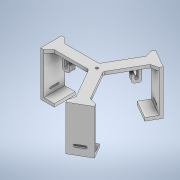
# Autodesk Inventor part: CalibrationRig_ver2
Saved by Autodesk Inventor 2022 (Build 260153000, 153)
## iProperties
Created: 2022-04-08
Part Number: CalibrationRig_ver2
Material: Generic
Document SubType Name: Modeling
Designer: victo
Density: 1 g/cm^3
Appearance: Default
Author: victo
Autodesk Inventor part; units mm, degrees
ref_plane "YZ Plane" through (0, 0, 0) normal (1, 0, 0) x (0, 1, 0)
ref_plane "XZ Plane" through (0, 0, 0) normal (0, 1, 0) x (-1, 0, 0)
ref_plane "XY Plane" through (0, 0, 0) normal (0, 0, 1) x (1, 0, 0)
sketch "Sketch1" plane through (0, 0, 0) normal (0, 1, 0) x (-1, 0, 0)
  line L0 (0, 0) -> (-20, 0)
  line L1 (0, 80) -> (-20, 80)
  line L2 (-20, 80) -> (-20, 120)
  line L3 (-20, 120) -> (0, 120)
  line L4 (0, 120) -> (6, 120)
  line L5 (6, 120) -> (6, 80)
  line L6 (6, 80) -> (0, 80)
  line L7 (-105.746, 18.9475) -> (-108.746, 13.7513)
  line L8 (-108.746, 13.7513) -> (-143.3871, 33.7513)
  line L9 (-143.3871, 33.7513) -> (-130.3871, 56.268)
  line L10 (-95.746, 36.268) -> (-108.746, 13.7513)
  line L11 (-95.746, 36.268) -> (-130.3871, 56.268)
  line L12 (-140.3871, 161.0525) -> (-143.3871, 166.2487)
  line L13 (-143.3871, 166.2487) -> (-108.746, 186.2487)
  line L14 (-108.746, 186.2487) -> (-95.746, 163.732)
  line L15 (-130.3871, 143.732) -> (-143.3871, 166.2487)
  line L16 (-130.3871, 143.732) -> (-95.746, 163.732)
  dimension "d12" = 40
  dimension "d13" = 6
  dimension "d15" = 6
  dimension "d16" = 40
  dimension "d18" = 6
  dimension "d19" = 40
  constraints: 34 end point, 2 horizontal, 2 perpendicular, 2 point on line, 1 collinear, 1 parallel, 1 vertical
  measures "d12" distance of L1.end L2.end
  measures "d13" distance of L3.end L4.end
  measures "d15" distance of L7.start L7.end
  measures "d16" distance of L7.end L8.end
  measures "d18" distance of L12.start L12.end
  measures "d19" distance of L12.end L13.end
extrude "Extrusion1" add sketch "Sketch1" along normal blind 6
sketch "Sketch2" plane through (0, 6, 0) normal (0, 1, 0) x (1, 0, 0)
  line L0 (-6, -80) -> (-6, -120) projected
  line L1 (20, -80) -> (-6, -80) projected
  line L2 (-6, -120) -> (0, -120)
  line L3 (0, -120) -> (0, -80)
  line L4 (0, -80) -> (-6, -80)
  line L5 (-6, -80) -> (-6, -120)
  line L6 (143.3871, -166.2487) -> (130.3871, -143.732) projected
  line L7 (95.746, -163.732) -> (108.746, -186.2487) projected
  line L8 (143.3871, -166.2487) -> (108.746, -186.2487)
  line L9 (108.746, -186.2487) -> (105.746, -181.0525)
  line L10 (105.746, -181.0525) -> (140.3871, -161.0525)
  line L11 (140.3871, -161.0525) -> (143.3871, -166.2487)
  line L12 (130.3871, -56.268) -> (143.3871, -33.7513) projected
  line L13 (143.3871, -33.7513) -> (108.746, -13.7513)
  line L14 (108.746, -13.7513) -> (105.746, -18.9475)
  line L15 (108.746, -13.7513) -> (95.746, -36.268) projected
  line L16 (143.3871, -33.7513) -> (108.746, -13.7513) projected
  line L17 (105.746, -18.9475) -> (140.3871, -38.9475)
  line L18 (143.3871, -33.7513) -> (140.3871, -38.9475)
  point P0 (0, 0)
  dimension "d22" = 6
  dimension "d23" = 6
  constraints: 24 end point, 8 perpendicular, 4 point on line, 2 parallel, 1 horizontal
  measures "d22" distance of L7.end L9.end
  measures "d23" distance of L13.end L14.end
extrude "Extrusion2" add sketch "Sketch2" along normal blind 80
sketch "Sketch3" plane through (0, 6, 120) normal (1, 0, 0) x (0, 0, -1)
  line L0 (0, 80) -> (40, 80) projected
  line L1 (40, -6) -> (40, 80) projected
  line L2 (0, 80) -> (40, 80)
  line L3 (40, 80) -> (40, 74)
  line L4 (40, 74) -> (0, 74)
  line L5 (0, 74) -> (0, 80)
  point P0 (120, -6)
  dimension "d26" = 6
  constraints: 8 end point, 2 parallel, 1 horizontal, 1 perpendicular, 1 point on line
  measures "d26" distance of L2.end L3.end
extrude "Extrusion3" add sketch "Sketch3" along normal blind 10
sketch "Sketch4" plane through (140.3871, 6, 38.9475) normal (-0.5, 0, 0.8660254) x (0.8660254, 0, 0.5)
  line L0 (0, 80) -> (-40, 80) projected
  line L1 (0, -6) -> (0, 80) projected
  line L2 (-40, 80) -> (0, 80)
  line L3 (0, 80) -> (0, 74)
  line L4 (0, 74) -> (-40, 74)
  line L5 (-40, 74) -> (-40, 80)
  point P0 (-141.0525, -6)
  dimension "d29" = 6
  constraints: 8 end point, 2 parallel, 1 horizontal, 1 perpendicular, 1 point on line
  measures "d29" distance of L2.end L3.end
extrude "Extrusion4" add sketch "Sketch4" along normal blind 10
sketch "Sketch5" plane through (105.746, 6, 181.0525) normal (-0.5, 0, -0.8660254) x (-0.8660254, 0, 0.5)
  line L0 (-40, 80) -> (0, 80) projected
  line L1 (0, 0) -> (0, 80) projected
  line L2 (-40, 80) -> (0, 80)
  line L3 (0, 80) -> (0, 74)
  line L4 (0, 74) -> (-40, 74)
  line L5 (-40, 74) -> (-40, 80)
  point P0 (1.0525, -6)
  dimension "d32" = 6
  constraints: 8 end point, 2 parallel, 1 horizontal, 1 perpendicular, 1 point on line
  measures "d32" distance of L2.end L3.end
extrude "Extrusion5" add sketch "Sketch5" along normal blind 10
chamfer "Chamfer1" distance 10 angle 45 6 edges at (100.746, 83, 27.6077) (135.3871, 83, 47.6077) (135.3871, 83, 152.3923) (100.746, 83, 172.3923) (10, 83, 120) (10, 83, 80)
sketch "Sketch6" plane through (135.3871, 6, 47.6077) normal (-0.5, 0, 0.8660254) x (0.8660254, 0, 0.5)
  line L0 (-30, 74) -> (-10, 74) projected
  line L1 (-10, 80) -> (-10, 74) projected
  line L2 (-30, 74) -> (-10, 74)
  line L3 (-10, 74) -> (-10, 80)
  line L4 (-10, 80) -> (-30, 80)
  line L5 (-30, 80) -> (-30, 74)
  point P0 (-141.0525, -6)
  constraints: 8 end point, 2 parallel, 1 horizontal, 1 perpendicular
extrude "Extrusion6" add sketch "Sketch6" along normal blind 90
sketch "Sketch7" plane through (10, 6, 120) normal (1, 0, 0) x (0, 0, -1)
  line L0 (10, 80) -> (0, 80) projected
  line L1 (30, 74) -> (40, 74) projected
  line L2 (10, 80) -> (30, 80)
  line L3 (30, 80) -> (30, 74)
  line L4 (30, 74) -> (10, 74)
  line L5 (10, 74) -> (10, 80)
  point P0 (120, -6)
  constraints: 8 end point, 2 parallel, 1 horizontal, 1 perpendicular
extrude "Extrusion7" add sketch "Sketch7" along normal through all
sketch "Sketch8" plane through (100.746, 6, 172.3923) normal (-0.5, 0, -0.8660254) x (-0.8660254, 0, 0.5)
  line L0 (-30, 80) -> (-40, 80) projected
  line L1 (-30, 74) -> (-10, 74) projected
  line L2 (-30, 80) -> (-10, 80)
  line L3 (-10, 80) -> (-10, 74)
  line L4 (-10, 74) -> (-30, 74)
  line L5 (-30, 74) -> (-30, 80)
  point P0 (1.0525, -6)
  constraints: 8 end point, 2 parallel, 1 horizontal, 1 perpendicular
extrude "Extrusion8" add sketch "Sketch8" along normal up to next
sketch "Sketch9" plane through (0, 86, 0) normal (0, 1, 0) x (1, 0, 0)
  line L0 (93.5914, -100) -> (113.5914, -100) construction
  line L1 (76.2709, -110) -> (64.7239, -110)
  line L2 (81.7268, -120.55) -> (64.4063, -110.55) projected
  line L3 (64.7239, -110) -> (64.4063, -110.55)
  line L4 (64.4063, -110.55) -> (81.7268, -120.55)
  line L5 (81.7268, -120.55) -> (82.0444, -120)
  line L6 (82.0444, -120) -> (76.2709, -110)
  point P0 (0, 0)
  dimension "d44" = 20
  constraints: 12 end point, 2 perpendicular, 1 collinear, 1 horizontal
  measures "d44" distance of L0.start L1.start
extrude "Extrusion9" cut sketch "Sketch9" against normal blind 10
sketch "Sketch10" plane through (0, 86, 0) normal (0, 1, 0) x (1, 0, 0)
  line L0 (126.7268, -157.3923) -> (93.5914, -100) projected
  line L1 (143.3871, -33.7513) -> (108.746, -13.7513) projected
  circle A0 centre (82.0444, -100) radius 2.5
  point P0 (0, 0)
  point P1 (76.2709, -110)
  dimension "d48" = 5
  constraints: 1 centre point
  measures "d48" diameter of A0
extrude "Extrusion10" cut sketch "Sketch10" against normal blind 10
fillet "Fillet1" radius 5 3 edges at (76.2709, 83, 110) (76.2709, 83, 90) (93.5914, 83, 100)
sketch "Sketch11" plane through (0, 80, 80) normal (0, -1, 0) x (1, 0, 0)
  line L0 (73.3841, 30) -> (10, 30) projected
  line L1 (20, 20) -> (20, 25)
  line L2 (20, 25) -> (25, 25)
  line L3 (25, 25) -> (25, 15)
  line L4 (25, 15) -> (20, 15)
  line L5 (20, 15) -> (20, 20)
  point P0 (0, -80)
  dimension "d54" = 5
  dimension "d55" = 10
  constraints: 10 end point, 3 perpendicular, 2 vertical
  measures "d54" distance of L1.end L2.end
  measures "d55" distance of L2.end L3.end
extrude "Extrusion11" add sketch "Sketch11" along normal blind 25
sketch "Sketch12" plane through (25, 80, 105) normal (1, 0, 0) x (0, 0, -1)
  line L0 (10, -25) -> (0, -25) projected
  line L1 (10, 0) -> (10, -25) projected
  line L2 (0, -25) -> (10, -25)
  line L3 (10, -25) -> (10, -20)
  line L4 (10, -20) -> (0, -20)
  line L5 (0, -20) -> (0, -25)
  point P0 (105, -80)
  dimension "d58" = 5
  constraints: 8 end point, 2 parallel, 1 horizontal, 1 perpendicular, 1 point on line
  measures "d58" distance of L3.end L2.end
extrude "Extrusion12" add sketch "Sketch12" along normal blind 10
sketch "Sketch13" plane through (25, 60, 105) normal (0, 1, 0) x (1, 0, 0)
  line L0 (0, 0) -> (10, 0) projected
  line L1 (0, 10) -> (10, 10) projected
  line L2 (10, 0) -> (5, 0)
  line L3 (5, 0) -> (5, 10)
  line L4 (5, 10) -> (10, 10)
  line L5 (10, 10) -> (10, 0)
  point P0 (-25, 105)
  constraints: 8 end point, 2 parallel, 1 horizontal, 1 midpoint, 1 perpendicular
extrude "Extrusion13" add sketch "Sketch13" along normal blind 10
fillet "Fillet2" radius 2.5 2 edges at (25, 60, 100) (30, 60, 100)
fillet "Fillet3" radius 5 2 edges at (20, 55, 100) (35, 55, 100)
fillet "Fillet4" radius 1 2 edges at (30, 70, 100) (35, 70, 100)
sketch "Sketch14" plane through (0, 80, 80) normal (0, -1, 0) x (1, 0, 0)
  line L0 (105.746, -61.0525) -> (109.4063, -47.3923) projected
  line L1 (109.4063, -47.3923) -> (118.0666, -42.3923)
  line L2 (109.4063, -47.3923) -> (77.7142, 7.5) projected
  line L3 (118.0666, -42.3923) -> (113.0666, -33.732)
  line L4 (113.0666, -33.732) -> (108.7364, -36.232)
  line L5 (108.7364, -36.232) -> (106.2364, -31.9019)
  line L6 (106.2364, -31.9019) -> (114.8967, -26.9019)
  line L7 (114.8967, -26.9019) -> (117.3967, -31.232)
  line L8 (117.3967, -31.232) -> (113.0666, -33.732)
  point P0 (0, -80)
  dimension "d66" = 10
  dimension "d67" = 10
  dimension "d68" = 5
  dimension "d69" = 5
  dimension "d70" = 10
  dimension "d71" = 5
  constraints: 14 end point, 5 perpendicular
  measures "d66" distance of L0.end L1.end
  measures "d67" distance of L1.end L3.end
  measures "d68" distance of L3.end L4.end
  measures "d69" distance of L4.end L5.end
  measures "d70" distance of L5.end L6.end
  measures "d71" distance of L6.end L7.end
extrude "Extrusion14" add sketch "Sketch14" along normal blind 25
sketch "Sketch15" plane through (106.2364, 55, 48.0981) normal (-0.5, 0, 0.8660254) x (0.8660254, 0, 0.5)
  line L0 (10, 25) -> (10, 0) projected
  line L1 (0, 0) -> (10, 0)
  line L2 (10, 0) -> (10, 5)
  line L3 (10, 5) -> (0, 5)
  line L4 (0, 5) -> (0, 0)
  point P0 (-116.0525, -55)
  dimension "d74" = 5
  constraints: 8 end point, 2 parallel, 1 horizontal, 1 perpendicular, 1 point on line
  measures "d74" distance of L2.end L1.end
extrude "Extrusion15" add sketch "Sketch15" along normal blind 10
sketch "Sketch16" plane through (106.2364, 60, 48.0981) normal (0, 1, 0) x (0.8660254, 0, 0.5)
  line L0 (10, 0) -> (10, -10) projected
  line L1 (0, 0) -> (0, -10) projected
  line L2 (10, -10) -> (0, -10)
  line L3 (0, -10) -> (0, -5)
  line L4 (0, -5) -> (10, -5)
  line L5 (10, -5) -> (10, -10)
  point P0 (-116.0525, -11.464)
  point P1 (0, -10)
  point P2 (10, -5)
  dimension "d77" = 5
  constraints: 8 end point, 2 parallel, 1 horizontal, 1 midpoint, 1 perpendicular
  measures "d77" distance of L2.end L3.end
extrude "Extrusion16" add sketch "Sketch16" along normal blind 10
sketch "Sketch17" plane through (0, 80, 80) normal (0, -1, 0) x (1, 0, 0)
  line L0 (140.3871, 81.0525) -> (126.7268, 77.3923) projected
  line L1 (109.4063, 87.3923) -> (105.746, 101.0525) projected
  line L2 (126.7268, 77.3923) -> (109.4063, 87.3923)
  line L3 (118.0666, 82.3923) -> (113.0666, 73.732)
  line L4 (113.0666, 73.732) -> (117.3967, 71.232)
  line L5 (117.3967, 71.232) -> (114.8967, 66.9019)
  line L6 (114.8967, 66.9019) -> (106.2364, 71.9019)
  line L7 (106.2364, 71.9019) -> (108.7364, 76.232)
  line L8 (108.7364, 76.232) -> (113.0666, 73.732)
  point P0 (0, -80)
  dimension "d80" = 10
  dimension "d81" = 5
  dimension "d82" = 5
  constraints: 14 end point, 5 perpendicular, 1 midpoint, 1 point on line
  measures "d80" distance of L3.start L3.end
  measures "d81" distance of L3.end L4.end
  measures "d82" distance of L4.end L5.end
extrude "Extrusion17" add sketch "Sketch17" along normal blind 25
sketch "Sketch18" plane through (114.8967, 55, 146.9019) normal (-0.5, 0, -0.8660254) x (-0.8660254, 0, 0.5)
  line L0 (10, 0) -> (0, 0) projected
  line L1 (10, 25) -> (10, 0) projected
  line L2 (0, 0) -> (10, 0)
  line L3 (10, 0) -> (10, 5)
  line L4 (10, 5) -> (0, 5)
  line L5 (0, 5) -> (0, 0)
  point P0 (26.0525, -55)
  dimension "d85" = 5
  constraints: 8 end point, 2 parallel, 1 horizontal, 1 perpendicular, 1 point on line
  measures "d85" distance of L3.end L2.end
extrude "Extrusion18" add sketch "Sketch18" along normal blind 10
sketch "Sketch19" plane through (106.2364, 60, 151.9019) normal (0, 1, 0) x (0.8660254, 0, -0.5)
  line L0 (0, 0) -> (0, 10) projected
  line L1 (10, 10) -> (0, 10)
  line L2 (0, 10) -> (0, 5)
  line L3 (0, 5) -> (10, 5)
  line L4 (10, 5) -> (10, 10)
  point P0 (-16.0525, 184.6691)
  dimension "d88" = 5
  constraints: 8 end point, 2 parallel, 1 horizontal, 1 midpoint, 1 perpendicular
  measures "d88" distance of L2.end L1.end
extrude "Extrusion19" add sketch "Sketch19" along normal blind 10
fillet "Fillet5" radius 1 4 edges at (108.0666, 70, 145.0717) (105.5666, 70, 140.7416) (108.0666, 70, 54.9283) (105.5666, 70, 59.2584)
fillet "Fillet6" radius 2.5 4 edges at (110.5666, 60, 50.5981) (108.0666, 60, 54.9283) (110.5666, 60, 149.4019) (108.0666, 60, 145.0717)
fillet "Fillet7" radius 5 4 edges at (113.0666, 55, 153.732) (105.5666, 55, 140.7416) (105.5666, 55, 59.2584) (113.0666, 55, 46.268)
sketch "Sketch20" plane through (143.3871, 0, 166.2487) normal (0.5, 0, 0.8660254) x (0.8660254, 0, -0.5)
  line L0 (-40, 0) -> (0, 0) projected
  circle A0 centre (-27.5, 16) radius 2.5
  circle A1 centre (-12.5, 16) radius 2.5
  line L1 (-27.5, 16) -> (-27.5, 18.5)
  line L2 (-12.5, 18.5) -> (-27.5, 18.5)
  line L3 (-27.5, 13.5) -> (-12.5, 13.5)
  point P0 (-41.0525, 0)
  dimension "d97" = 5
  dimension "d98" = 5
  constraints: 6 end point, 4 point on circle, 2 centre point, 1 perpendicular, 1 point on line, 1 tangent, 1 vertical
  measures "d97" diameter of A0
  measures "d98" diameter of A1
extrude "Extrusion20" cut sketch "Sketch20" against normal blind 3
sketch "Sketch21" plane through (141.8871, 0, 163.6506) normal (0.5, 0, 0.8660254) x (0.8660254, 0, -0.5)
  line L0 (-27.5, 18.5) -> (-12.5, 18.5) projected
  arc A0 (-27.5, 18.5) -> (-27.5, 13.5) centre (-27.5, 16) ccw projected
  arc A1 (-27.5, 17.25) -> (-27.5, 14.75) centre (-27.5, 16) ccw
  line L1 (-27.5, 17.25) -> (-12.5, 17.25)
  arc A2 (-12.5, 14.75) -> (-12.5, 17.25) centre (-12.5, 16) ccw
  line L2 (-12.5, 14.75) -> (-27.5, 14.75)
  point P0 (-41.0525, 0)
  dimension "d101" = 2.5
  dimension "d102" = 15
  constraints: 4 end point, 4 point on circle, 2 centre point, 1 coincident, 1 horizontal, 1 tangent
  measures "d101" diameter of A1
  measures "d102" distance of L1.start L1.end
extrude "Extrusion21" cut sketch "Sketch21" against normal blind 3
sketch "Sketch22" plane through (108.746, 0, 13.7513) normal (0.5, 0, -0.8660254) x (-0.8660254, 0, -0.5)
  line L0 (0, 0) -> (-40, 0) projected
  arc A0 (-12.5, 13.5) -> (-12.5, 18.5) centre (-12.5, 16) ccw
  arc A1 (-27.5, 18.5) -> (-27.5, 13.5) centre (-27.5, 16) ccw
  line L1 (-27.5, 18.5) -> (-12.5, 18.5)
  line L2 (-27.5, 13.5) -> (-12.5, 13.5)
  point P0 (101.0525, 0)
  dimension "d108" = 5
  dimension "d109" = 5
  constraints: 4 end point, 4 point on circle, 2 centre point, 2 tangent
  measures "d108" diameter of A0
  measures "d109" diameter of A1
extrude "Extrusion22" cut sketch "Sketch22" against normal blind 3
sketch "Sketch23" plane through (107.246, 0, 16.3494) normal (0.5, 0, -0.8660254) x (-0.8660254, 0, -0.5)
  arc A0 (-27.5, 18.5) -> (-27.5, 13.5) centre (-27.5, 16) ccw projected
  arc A1 (-27.5, 17.25) -> (-27.5, 14.75) centre (-27.5, 16) ccw
  line L0 (-27.5, 17.25) -> (-12.5, 17.25)
  arc A2 (-12.5, 14.75) -> (-12.5, 17.25) centre (-12.5, 16) ccw
  line L1 (-27.5, 14.75) -> (-12.5, 14.75)
  point P0 (101.0525, 0)
  dimension "d112" = 2.5
  dimension "d113" = 15
  constraints: 4 end point, 4 point on circle, 2 centre point, 2 tangent, 1 coincident, 1 horizontal
  measures "d112" diameter of A1
  measures "d113" distance of L0.start L0.end
extrude "Extrusion23" cut sketch "Sketch23" against normal blind 3
sketch "Sketch24" plane through (-6, 0, 80) normal (-1, 0, 0) x (0, 0, 1)
  line L0 (40, 0) -> (0, 0) projected
  arc A0 (27.5, 13.5) -> (27.5, 18.5) centre (27.5, 16) ccw
  arc A1 (12.5, 18.5) -> (12.5, 13.5) centre (12.5, 16) ccw
  line L1 (27.5, 18.5) -> (12.5, 18.5)
  line L2 (27.5, 13.5) -> (12.5, 13.5)
  point P0 (-80, 0)
  dimension "d119" = 5
  dimension "d120" = 5
  constraints: 4 end point, 4 point on circle, 2 centre point, 2 tangent
  measures "d119" diameter of A0
  measures "d120" diameter of A1
extrude "Extrusion24" cut sketch "Sketch24" against normal blind 3
sketch "Sketch25" plane through (-3, 0, 80) normal (-1, 0, 0) x (0, 0, 1)
  line L0 (12.5, 18.5) -> (27.5, 18.5) projected
  arc A0 (27.5, 13.5) -> (27.5, 18.5) centre (27.5, 16) ccw projected
  arc A1 (27.5, 14.5) -> (27.5, 17.5) centre (27.5, 16) ccw
  line L1 (27.5, 17.5) -> (12.5, 17.5)
  arc A2 (12.5, 17.5) -> (12.5, 14.5) centre (12.5, 16) ccw
  line L2 (12.5, 14.5) -> (27.5, 14.5)
  point P0 (-80, 0)
  dimension "d123" = 3
  constraints: 4 end point, 4 point on circle, 2 centre point, 1 coincident, 1 horizontal, 1 tangent
  measures "d123" diameter of A1
extrude "Extrusion25" cut sketch "Sketch25" against normal blind 3
body "Solid1"
